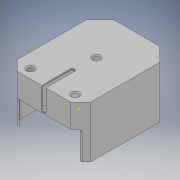
# Autodesk Inventor part: Kozhuh_Lock_Left
Saved by Autodesk Inventor 2017 (Build 210142000, 142)
## iProperties
Part Number: Kozhuh_Lock_Left
Material: Типовые
Document SubType Name: Modeling
Designer: yulia_000
Density: 1 g/cm^3
Appearance: По умолчанию
Author: yulia_000
## iProperties of the stored document Kozhuh_Lock_Right_3DПЕЧАТЬ.ipt
Part Number: Kozhuh_Lock_Right_3DПЕЧАТЬ
Material: Типовые
Document SubType Name: Modeling
Designer: Nikita
Density: 1 g/cm^3
Appearance: По умолчанию
Author: Nikita
Autodesk Inventor part; units mm, degrees
ref_plane "YZ Plane" through (0, 0, 0) normal (1, 0, 0) x (0, 1, 0)
ref_plane "XZ Plane" through (0, 0, 0) normal (0, 1, 0) x (-1, 0, 0)
ref_plane "XY Plane" through (0, 0, 0) normal (0, 0, 1) x (1, 0, 0)
sketch "Эскиз1" plane through (0, 0, 0) normal (0, 1, 0) x (-1, 0, 0)
  line L0 (11, 0) -> (49, 0)
  line L1 (60, -11) -> (60, -68.5)
  line L2 (51.5, -77) -> (8.5, -77)
  line L3 (0, -68.5) -> (0, -11)
  line L4 (60, -11) -> (49, 0)
  line L5 (60, -68.5) -> (51.5, -77)
  line L6 (8.5, -77) -> (0, -68.5)
  line L7 (0, -11) -> (11, 0)
  line L8 (61.2, -68.9971) -> (51.9971, -78.2)
  line L9 (51.9971, -78.2) -> (8.0029, -78.2)
  line L10 (8.0029, -78.2) -> (-1.2, -68.9971)
  line L11 (-1.2, -68.9971) -> (-1.2, -10.5029)
  line L12 (-1.2, -10.5029) -> (10.5029, 1.2)
  line L13 (10.5029, 1.2) -> (49.4971, 1.2)
  line L14 (49.4971, 1.2) -> (61.2, -10.5029)
  line L15 (61.2, -10.5029) -> (61.2, -68.9971)
  line L16 (31.75, -52) -> (28.25, -52)
  line L17 (28.25, -52) -> (28.25, -77)
  line L18 (28.25, -77) -> (31.75, -77)
  line L19 (31.75, -77) -> (31.75, -52)
  line L20 (31.75, -52) -> (28.25, -77) construction
  line L21 (28.25, -52) -> (31.75, -77) construction
  point P0 (0, 0)
  point P1 (60, -77)
  point P2 (60, 0)
  point P3 (0, -77)
  point P4 (30, -64.5)
  point P5 (30, -77)
  dimension "d8" = 60
  dimension "d9" = 77
  dimension "d10" = 11
  dimension "d11" = 11
  dimension "d12" = 8.5
  dimension "d13" = 8.5
  dimension "d14" = 8.5
  dimension "d15" = 8.5
  dimension "d16" = 11
  dimension "d17" = 11
  dimension "d18" = 1.2
  dimension "d51" = 3.5
  dimension "d52" = 25
  constraints: 44 end point, 8 point on line, 6 parallel, 4 midpoint, 3 perpendicular, 2 horizontal, 7 other
  measures "d8" distance of point (60, -77) point (0, -77)
  measures "d9" distance of point (60, 0) point (60, -77)
  measures "d10" distance of L1.start point (60, 0)
  measures "d11" distance of L0.end point (60, 0)
  measures "d12" distance of L1.end point (60, -77)
  measures "d13" distance of L2.start point (60, -77)
  measures "d14" distance of L2.end point (0, -77)
  measures "d15" distance of L3.start point (0, -77)
  measures "d16" distance of L3.end point (0, 0)
  measures "d17" distance of L0.start point (0, 0)
  measures "d18" distance between parallel lines of L1 L15
  measures "d51" distance of L18.end L17.end
  measures "d52" distance of L17.end L16.end
extrude "Выдавливание1" add sketch "Эскиз1" against normal blind 1 contours L0 L4 L1 L5 L2 L19 L16 L17 L6 L3 L7 | L17 L16 L19 L2 | L8 L9 L10 L11 L12 L13 L14 L15
extrude "Выдавливание2" add sketch "Эскиз1" along normal blind 43
fillet "Сопряжение1" radius 1 8 edges at (-60, 0, -39.75) (-55.75, 0, -72.75) (-30, 0, -77) (-4.25, 0, -72.75) (0, 0, -39.75) (-5.5, 0, -5.5) (-30, 0, 0) (-54.5, 0, -5.5)
extrude "Выдавливание3" add sketch "Эскиз1" along normal blind 18 separate body contours L17 L16 L19 L2
sketch "Эскиз2" plane through (-28.25, 0, -77) normal (0, 0, -1) x (-1, 0, 0)
  line L0 (0, 0) -> (3.5, 0) projected
  line L1 (3.5, 0) -> (3.5, 18) projected
  line L2 (0, 18) -> (3.5, 18) projected
  line L3 (0, 0) -> (0, 18) projected
  point P0 (-28.25, 0)
extrude "Выдавливание4" add sketch "Эскиз2" along normal blind 17 bodies 2
sketch "Эскиз3" plane through (0, 0, 0) normal (0, -1, 0) x (1, 0, 0)
  line L0 (-28.25, -52) -> (-28.25, -94) projected
  line L1 (-31.75, -52) -> (-28.25, -52) projected
  line L2 (-31.75, -52) -> (-31.75, -94) projected
  line L3 (-28.25, -94) -> (-31.75, -94) projected
  point P0 (0, 0)
extrude "Выдавливание5" add sketch "Эскиз3" along normal blind 18 bodies 2
combine bodies "Комбинировать1" operation type subtract main body 1 bodies to subtract 2
hole "Отверстие4" at (-49, -1, -70) direction (0, 1, 0) diameter 4.2 end through all countersink diameter 7 countersink angle 90 bodies 1
hole "Отверстие5" at (-11, -1, -70) direction (0, 1, 0) diameter 4.2 end through all countersink diameter 7 countersink angle 90 bodies 1
hole "Отверстие6" at (-29, -1, -34) direction (0, 1, 0) diameter 4.2 end through all countersink diameter 7 countersink angle 90 bodies 1
fillet "Сопряжение2" radius 1 16 edges at (-59.7071, 0.2929, -68.3787) (-60, 22, -68.5) (-51.3787, 0.2929, -76.7071) (-51.5, 22, -77) (-8.6213, 0.2929, -76.7071) (-8.5, 22, -77) (-0.2929, 0.2929, -68.3787) (0, 22, -68.5) (-0.2929, 0.2929, -11.1213) (0, 22, -11) (-11.1213, 0.2929, -0.2929) (-11, 22, 0) (-48.8787, 0.2929, -0.2929) (-49, 22, 0) (-59.7071, 0.2929, -11.1213) (-60, 22, -11)
fillet "Сопряжение3" radius 1 4 edges at (-31.75, -0.5, -52) (-28.25, -0.5, -52) (-28.25, 18, -77.6) (-31.75, 18, -77.6)
sketch "Эскиз4" plane through (-8.0029, 43, -78.2) normal (0, 0, -1) x (-1, 0, 0)
  line L0 (43.9941, 0) -> (43.9941, -44) projected
  line L1 (0, 0) -> (43.9941, 0) projected
  line L2 (0, 0) -> (0, -44) projected
  line L3 (43.9941, 0) -> (43.9941, -24)
  line L4 (43.9941, -24) -> (0, -24)
  line L5 (0, -24) -> (0, 0)
  line L6 (0.2042, 0) -> (-7.7101, 0) projected
  line L7 (0, 0) -> (43.9941, 0)
  line L8 (41.2899, 0) -> (51.7042, 0) projected
  point P0 (-8.0029, -43)
  dimension "d88" = 24
  constraints: 8 end point, 2 perpendicular, 2 point on line, 1 collinear
  measures "d88" distance of L0.start L3.end
extrude "Выдавливание6" add sketch "Эскиз4" against normal blind 5.5 separate body
sketch "Эскиз5" plane through (-51.9971, 19, -78.2) normal (-1, 0, 0) x (0, 0, 1)
  line L0 (0, 0) -> (0, 24) projected
  line L1 (0, 0) -> (5.5, 0) projected
  line L2 (5.5, 24) -> (5.5, 0) projected
  line L3 (0, 24) -> (5.5, 24) projected
  point P0 (78.2, -19)
extrude "Выдавливание7" add sketch "Эскиз5" along normal blind 10 bodies 3
sketch "Эскиз6" plane through (-8.0029, 19, -78.2) normal (1, 0, 0) x (0, 0, -1)
  line L0 (0, 24) -> (0, 0) projected
  line L1 (0, 24) -> (-5.5, 24) projected
  line L2 (-5.5, 0) -> (-5.5, 24) projected
  line L3 (0, 0) -> (-5.5, 0) projected
  point P0 (-78.2, -19)
extrude "Выдавливание8" add sketch "Эскиз6" along normal blind 10 bodies 3
combine bodies "Комбинировать2" operation type subtract main body 1 bodies to subtract 3
fillet "Сопряжение4" radius 2 2 edges at (-56.6485, 19, -72.7) (-3.3515, 19, -72.7)
sketch "Эскиз7" plane through (-61.2, -1, -68.9971) normal (-1, 0, 0) x (0, 0, 1)
  line L0 (58.4941, 0) -> (0, 0) projected
  line L1 (58.4941, 44) -> (58.4941, 0) projected
  line L2 (26.9941, 14) -> (29.9941, 14) construction
  line L3 (26.9941, 13) -> (29.9941, 13)
  line L4 (29.9941, 15) -> (26.9941, 15)
  arc A0 (26.9941, 15) -> (26.9941, 13) centre (26.9941, 14) ccw
  arc A1 (29.9941, 13) -> (29.9941, 15) centre (29.9941, 14) ccw
  point P0 (68.9971, 1)
  point P1 (28.4941, 14)
  dimension "d96" = 3
  dimension "d97" = 2
  dimension "d98" = 13
  dimension "d99" = 30
  constraints: 8 end point, 4 point on circle, 4 tangent, 2 centre point, 1 horizontal, 1 midpoint, 1 parallel
  measures "d96" distance of L2.start L2.end
  measures "d97" diameter of A1
  measures "d98" distance between parallel lines of L0 L3
  measures "d99" distance from line of L1 point (28.494, 14)
extrude "Выдавливание9" cut sketch "Эскиз7" against normal up to surface (1.2 mm away) bodies 1
sketch "Эскиз8" plane through (-8.0029, -1, -78.2) normal (0, 0, -1) x (-1, 0, 0)
  point P0 (-8.0029, 1)
sketch "Эскиз9" plane through (-8.0029, -1, -78.2) normal (0, 0, -1) x (-1, 0, 0)
  point P0 (-8.0029, 1)
sketch "Эскиз10" plane through (-8.0029, -1, -78.2) normal (0, 0, -1) x (-1, 0, 0)
  point P0 (-8.0029, 1)
sketch "Эскиз11" plane through (-51.9971, 19, -78.2) normal (0, 1, 0) x (1, 0, 0)
  line L0 (47.4941, -3.5) -> (45.7971, -3.5) projected
  line L1 (43.9941, 0) -> (47.4941, -3.5) projected
  line L2 (0, 0) -> (43.9941, 0) projected
  line L3 (-3.5, -3.5) -> (0, 0) projected
  line L4 (-1.8029, -3.5) -> (-3.5, -3.5) projected
  line L5 (0.2042, -1.4929) -> (-1.8029, -3.5) projected
  arc A0 (0.9113, -1.2) -> (0.2042, -1.4929) centre (0.9113, -2.2) ccw projected
  line L6 (43.0828, -1.2) -> (0.9113, -1.2) projected
  arc A1 (43.7899, -1.4929) -> (43.0828, -1.2) centre (43.0828, -2.2) ccw projected
  line L7 (45.7971, -3.5) -> (43.7899, -1.4929) projected
  line L8 (44.5941, -0.6) -> (-0.6, -0.6)
  line L9 (0, 0) -> (43.9941, 0) projected
  line L10 (21.9971, 0) -> (21.9971, -1.2)
  line L11 (21.2471, -1.2) -> (22.7471, -1.2) projected
  point P0 (51.9971, -78.2)
  point P1 (21.9971, -0.6)
  constraints: 4 end point, 4 midpoint, 2 point on line, 1 horizontal
extrude "Выдавливание10" cut sketch "Эскиз11" against normal up to surface (20 mm away) contours L8 L10 L2 L1 | L8 L3 L2 L10 bodies 1
equation "\"d13\" = d12"
